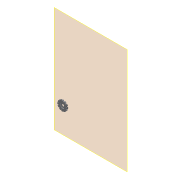
# Autodesk Inventor part: cellSTORM_screw_ring_adjuster
Saved by Autodesk Inventor 2019 (Build 230136000, 136)
## iProperties
Created: 2019-12-12
Part Number: cellSTORM_screw_ring_adjuster
Material: Generic
Document SubType Name: Modeling
Designer: diederichbenedict
Density: 1 g/cm^3
Appearance: Default
Author: diederichbenedict
Autodesk Inventor part; units mm, degrees
ref_plane "YZ Plane" through (0, 0, 0) normal (1, 0, 0) x (0, 1, 0)
ref_plane "XZ Plane" through (0, 0, 0) normal (0, 1, 0) x (-1, 0, 0)
ref_plane "XY Plane" through (0, 0, 0) normal (0, 0, 1) x (1, 0, 0)
ref_plane "Work Plane1" through (-89.269, -103.4593, 127.4153) normal (0, 0, 1) x (0, -1, 0)
sketch "Sketch1" plane through (-89.269, -103.4593, 127.4153) normal (0, 0, 1) x (0, -1, 0)
  circle A0 centre (44.9313, -45.255) radius 1.4 construction
  circle A1 centre (44.9313, -45.255) radius 1.7
  circle A2 centre (44.9313, -45.255) radius 6.7
  point P0 (-103.4593, 89.269)
  dimension "d0" = 0.3
  dimension "d1" = 5
  constraints: 2 centre point
  measures "d0" radial gap between concentric circles of A0 A1
  measures "d1" radial gap between concentric circles of A1 A2
extrude "Extrusion1" add sketch "Sketch1" along normal blind 2
sketch "Sketch2" plane through (-134.524, -148.3906, 129.4153) normal (0, 0, 1) x (1, 0, 0)
  circle A0 centre (0, 0) radius 1.7 projected
  circle A1 centre (0, 0) radius 6.7 projected
  line L0 (-6.7, 0) -> (-8.0802, 0)
  line L1 (-8.0802, 0) -> (-7.8365, -1.3818)
  line L2 (-7.8365, -1.3818) -> (-6.5982, -1.1634)
  circle A2 centre (0, 0) radius 6.7 projected
  line L3 (0, 0) -> (-6.5982, -1.1634)
  line L4 (0, 0) -> (-6.7, 0)
  line L5 (0, 0) -> (6.7, 0) construction
  line L6 (-8.0802, 0) -> (-7.8365, 1.3818)
  line L7 (-7.8365, 1.3818) -> (-6.5982, 1.1634)
  arc A3 (-6.5982, 1.1634) -> (-6.5982, -1.1634) centre (0, 0) ccw
  point P0 (134.524, 148.3906)
  dimension "d4" = 180
  dimension "d7" = 10
  constraints: 16 end point, 5 point on circle, 2 collinear, 2 horizontal, 2 symmetric about line, 1 centre point, 1 horizontal alignment, 1 perpendicular, 1 other
  measures "d4" angle of L4 L5
  measures "d7" angle of L3 L4
extrude "Extrusion2" add sketch "Sketch2" against normal up to surface (2 mm away) contours L0 L6 L7 A1 | A1 L2 L1 L0
pattern_circular "Circular Pattern1" count 12 over 360 about axis through (-134.524, -148.3906, 127.4153) along (0, 0, 1) of "Extrusion2"
sketch "Sketch3" plane through (-89.269, -103.4593, 129.4153) normal (0, 0, 1) x (1, 0, 0)
  circle A0 centre (-45.255, -44.9313) radius 2.45 projected
  line L0 (-42.7892, -48.1333) -> (-46.7952, -48.6677)
  line L1 (-46.7952, -48.6677) -> (-49.261, -45.4657)
  line L2 (-49.261, -45.4657) -> (-47.7208, -41.7292)
  line L3 (-47.7208, -41.7292) -> (-43.7148, -41.1948)
  line L4 (-43.7148, -41.1948) -> (-41.249, -44.3969)
  line L5 (-41.249, -44.3969) -> (-42.7892, -48.1333)
  point P0 (89.269, 103.4593)
  dimension "d11" = 7
  constraints: 12 end point, 1 coincident, 13 other
  measures "d11" distance between parallel lines of L0 L3
extrude "Extrusion3" cut sketch "Sketch3" against normal blind 1.5 contours A0 | L0 L1 L2 L3 L4 L5
body "Solid1"
